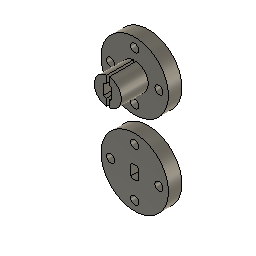
stepperFlangeBracket (Autodesk Fusion 360 design; units mm, degrees)
Autodesk Fusion 360 part; units mm, degrees
sketch "Sketch1" plane through (0, 0, 0) normal (0, 1, 0) x (1, 0, 0) in component "laserCutExample"
  line L0 (0, 0) -> (0, 2.45) construction
  line L1 (-1.5, -1.9371) -> (-1.5, 1.9371)
  line L2 (1.5, -1.9371) -> (1.5, 1.9371)
  arc A0 (-1.5, -1.9371) -> (1.5, -1.9371) centre (0, 0) ccw
  arc A1 (1.5, 1.9371) -> (-1.5, 1.9371) centre (0, 0) ccw
  circle A2 centre (0, 0) radius 12.5
  circle A3 centre (0, -9) radius 1.5
  circle A4 centre (9, 0) radius 1.5
  circle A5 centre (0, 9) radius 1.5
  circle A6 centre (-9, 0) radius 1.5
  dimension "d1" = 4.9
  dimension "d2" = 3
  dimension "d3" = 3
  dimension "d4" = 9
  dimension "d6" = 360
  dimension "d14" = 25
  constraint coincident L0.start A0.centre
  constraint coincident L0.end A1
  constraint vertical L0
  constraint parallel L0 L1
  constraint parallel L1 L2
  constraint symmetric L0 L1 L2
  constraint concentric A0 A1
  constraint concentric A0 A2
  constraint horizontal A4.centre A6.centre
  measures "d1" diameter of A0
  measures "d2" distance of L1 L2
  measures "d3" diameter of A3
  measures "d4" distance of L0.start A3.centre
  measures "d14" diameter of A2
extrude "Extrude1" add sketch "Sketch1" along normal blind 5 makes body 1 in component "laserCutExample"
sketch "Sketch1 (2)" plane through (0, 0, 0) normal (0, 1, 0) x (1, 0, 0) in component "3dPrintExample"
  line L0 (0, 0) -> (0, 2.45) construction
  line L1 (-1.5, -1.9371) -> (-1.5, 1.9371)
  line L2 (1.5, -1.9371) -> (1.5, 1.9371)
  arc A0 (-1.5, -1.9371) -> (1.5, -1.9371) centre (0, 0) ccw
  arc A1 (1.5, 1.9371) -> (-1.5, 1.9371) centre (0, 0) ccw
  circle A2 centre (0, 0) radius 12.5
  circle A3 centre (0, -9) radius 1.5
  circle A4 centre (9, 0) radius 1.5
  circle A5 centre (0, 9) radius 1.5
  circle A6 centre (-9, 0) radius 1.5
  dimension "d1_1" = 4.9
  dimension "d2_1" = 3
  dimension "d3_1" = 3
  dimension "d4_1" = 9
  dimension "d6_1" = 360
  dimension "d11" = 25
  constraint coincident L0.start A0.centre
  constraint coincident L0.end A1
  constraint vertical L0
  constraint parallel L0 L1
  constraint parallel L1 L2
  constraint symmetric L0 L1 L2
  constraint concentric A0 A1
  constraint concentric A0 A2
  constraint horizontal A4.centre A6.centre
  measures "d1_1" diameter of A0
  measures "d2_1" distance of L1 L2
  measures "d3_1" diameter of A3
  measures "d4_1" distance of L0.start A3.centre
  measures "d11" diameter of A2
extrude "Extrude1'" add sketch "Sketch1 (2)" along normal blind 5 separate body makes body 2 in component "3dPrintExample"
sketch "Sketch2" plane through (0, 0, 0) normal (0, -1, 0) x (1, 0, 0) in component "3dPrintExample"
  arc A0 (1.5, 1.9371) -> (-1.5, 1.9371) centre (0, 0) ccw
  line L0 (1.5, 1.9371) -> (1.5, -1.9371)
  arc A1 (-1.5, -1.9371) -> (1.5, -1.9371) centre (0, 0) ccw
  line L1 (-1.5, -1.9371) -> (-1.5, 1.9371)
  circle A2 centre (0, -9) radius 1.5
  circle A3 centre (-9, 0) radius 1.5
  circle A4 centre (0, 9) radius 1.5
  circle A5 centre (9, 0) radius 1.5
  circle A6 centre (0, 0) radius 12.5
  circle A7 centre (0, 0) radius 5
  line L2 (-0.5, -5) -> (0.5, -5)
  line L3 (0.5, -5) -> (0.5, 5)
  line L4 (0.5, 5) -> (-0.5, 5)
  line L5 (-0.5, 5) -> (-0.5, -5)
  line L6 (-0.5, -5) -> (0.5, 5) construction
  line L7 (0.5, -5) -> (-0.5, 5) construction
  dimension "d12" = 10
  dimension "d13" = 1
  constraint concentric A0 A7
  constraint horizontal L2
  constraint perpendicular L2 L3
  constraint parallel L2 L4
  constraint parallel L3 L5
  constraint coincident L6 A0.centre
  constraint coincident L7 A0.centre
  constraint coincident A0.centre A1.centre
  constraint tangent A7 L2
  measures "d12" diameter of A7
  measures "d13" distance of L3 L5
extrude "Extrude2" add sketch "Sketch2" along normal blind 10 contours A0 L0 A1 A7 L3 | A0 A1 L1 A7 L5 bodies 2 in component "3dPrintExample"
component "laserCutExample" placed x (1, 0, 0) y (0, 1, 0) z (0, 0, 1) at (0, 0, 0)
component "3dPrintExample" placed x (1, 0, 0) y (0, 1, 0) z (0, 0, 1) at (0, 0, 30.9564)
